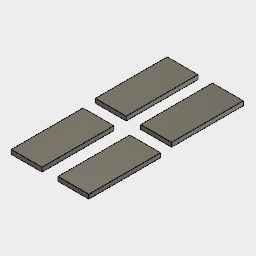
Box Hinges v5 (Autodesk Fusion 360 design; units mm, degrees)
Autodesk Fusion 360 part; units mm, degrees
sketch "Sketch1" plane through (0, 0, 0) normal (0, 1, 0) x (1, 0, 0)
  line L0 (0, 0) -> (-21.5, 0)
  line L1 (-21.5, 0) -> (-21.5, 50)
  line L2 (-21.5, 50) -> (0, 50)
  line L3 (0, 50) -> (0, 0)
  line L4 (-21.5, 25) -> (0, 25)
  line L5 (10, 0) -> (31.5, 0)
  line L6 (31.5, 0) -> (31.5, 50)
  line L7 (31.5, 50) -> (10, 50)
  line L8 (10, 50) -> (10, 0)
  line L9 (-20, -10) -> (1.5, -10)
  line L10 (1.5, -10) -> (1.5, -60)
  line L11 (1.5, -60) -> (-20, -60)
  line L12 (-20, -60) -> (-20, -10)
  line L13 (12.5136, -10) -> (34.0136, -10)
  line L14 (34.0136, -10) -> (34.0136, -60)
  line L15 (34.0136, -60) -> (12.5136, -60)
  line L16 (12.5136, -60) -> (12.5136, -10)
  line L17 (10, 25) -> (31.5, 25)
  line L18 (34.0136, -35) -> (12.5136, -35)
  line L19 (-20, -35) -> (1.5, -35)
  dimension "d1" = 21.5
  dimension "d2" = 50
  dimension "d3" = 25
  dimension "d4" = 21.5
  dimension "d5" = 21.5
  dimension "d6" = 21.5
  dimension "d7" = 50
  dimension "d8" = 25
  constraint horizontal L0
  constraint vertical L1
  constraint horizontal L2
  constraint vertical L3
  constraint coincident L1
  constraint perpendicular L1 L4
  constraint coincident L3
  constraint horizontal L5
  constraint vertical L6
  constraint horizontal L7
  constraint vertical L8
  constraint horizontal L9
  constraint vertical L10
  constraint horizontal L11
  constraint vertical L12
  constraint horizontal L13
  constraint vertical L14
  constraint horizontal L15
  constraint vertical L16
  constraint midpoint L8
  constraint midpoint L6
  constraint midpoint L14
  constraint midpoint L16
  constraint midpoint L12
  constraint midpoint L10
  measures "d3" distance of L0 L4
  measures "d8" distance of L11 L19
extrude "Extrude1" add sketch "Sketch1" along normal blind 3 makes body 1 at (24.3333, 0, -16.6667) makes body 2 at (26.8469, 0, 43.3333) makes body 3 at (-7.1667, 0, -16.6667) makes body 4 at (-12.8333, 0, 26.6667)
